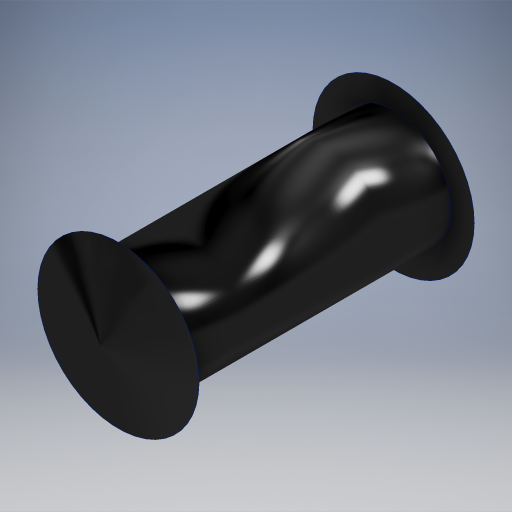
# Autodesk Inventor part: link7
Saved by Autodesk Inventor 2024.1 (Build 281209000, 209)
## iProperties
Created: 2023-09-09
Part Number: link7
Material: Aluminum 6061
Document SubType Name: Modeling
Designer: Camilo
Density: 2.7 g/cm^3
Appearance: Aluminum - Flat
Mass: 0.0921726 g
Surface Area: 0.787299 cm^2
Volume: 0.034138 cm^3
Author: Camilo
Autodesk Inventor part; units mm, degrees
ref_plane "YZ Plane" through (0, 0, 0) normal (1, 0, 0) x (0, 1, 0)
ref_plane "XZ Plane" through (0, 0, 0) normal (0, 1, 0) x (-1, 0, 0)
ref_plane "XY Plane" through (0, 0, 0) normal (0, 0, 1) x (1, 0, 0)
sketch "Sketch2" plane through (0, 0, 0) normal (0, 0, 1) x (1, 0, 0)
  circle A0 centre (0, 0) radius 1.25
  dimension "d44" = 2.5
  constraints: 1 centre point, 1 coincident
  measures "d44" diameter of A0
extrude "Extrusion8" add sketch "Sketch2" along normal mid plane 6
sketch "Sketch3" plane through (0, 0, 3) normal (0, 0, 1) x (1, 0, 0)
  circle A0 centre (0, 0) radius 1.75
  dimension "d47" = 3.5
  constraints: 1 centre point, 1 coincident
  measures "d47" diameter of A0
sketch "Sketch4" plane through (0, 0, 0) normal (0, 1, 0) x (-1, 0, 0)
  line L0 (1.25, 3) -> (-1.25, 3) projected
  line L1 (0, 3) -> (0, 3.4)
  arc A0 (0, 3.4) -> (-1.761, 3) centre (0.2088, -1.5956) ccw
  line L2 (0, 3) -> (-1.761, 3)
  point P0 (0, 0)
  dimension "d48" = 0.4
  dimension "d49" = 5
  constraints: 4 end point, 2 point on circle, 1 centre point, 1 horizontal, 1 midpoint, 1 vertical
  measures "d48" distance of L1.start L1.end
  measures "d49" radius of A0
revolve "Revolution1" add sketch "Sketch4" angle 360 about axis through (0, 0, 3) along (0, 0, 1)
mirror "Mirror1" about plane through (0, 0, 0) normal (0, 0, 1) of "Revolution1"
body "Solid3"
